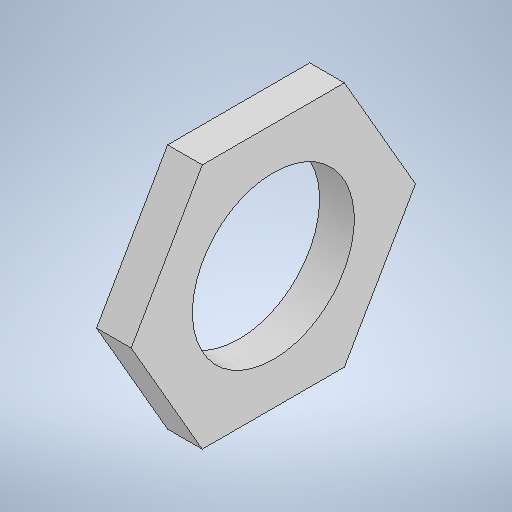
# Autodesk Inventor part: CH-2(Gearbox_Output_Spacer)
Saved by Autodesk Inventor 2025.1 (Build 291241020, 241B)
## iProperties
Created: 2024-10-02
Part Number: CH-2(Gearbox_Output_Spacer)
Material: Generic
Document SubType Name: Modeling
Designer: aidan
Density: 1 g/cm^3
Appearance: Default
Author: aidan
Autodesk Inventor part; units mm, degrees
ref_plane "YZ Plane" through (0, 0, 0) normal (1, 0, 0) x (0, 1, 0)
ref_plane "XZ Plane" through (0, 0, 0) normal (0, 1, 0) x (-1, 0, 0)
ref_plane "XY Plane" through (0, 0, 0) normal (0, 0, 1) x (1, 0, 0)
sketch "Sketch1" plane through (0, 0, 0) normal (1, 0, 0) x (0, 1, 0)
  circle A0 centre (0, 0) radius 7.112
  circle A1 centre (0, 0) radius 12.7
  line L0 (10.8193, 6.6508) -> (10.8193, -6.6508)
  line L1 (-0.3501, 12.6952) -> (11.1694, 6.0444)
  line L2 (-11.1694, 6.0444) -> (0.3501, 12.6952)
  line L3 (-10.8193, -6.6508) -> (-10.8193, 6.6508)
  line L4 (0.3501, -12.6952) -> (-11.1694, -6.0444)
  line L5 (11.1694, -6.0444) -> (-0.3501, -12.6952)
  point P0 (0, -12.4931)
  point P1 (10.8193, -6.2465)
  point P2 (10.8193, 6.2465)
  point P3 (0, 12.4931)
  point P4 (-10.8193, 6.2465)
  point P5 (-10.8193, -6.2465)
  dimension "d0" = 14.224
  dimension "d1" = 25.4
  dimension "d6" = 360
  constraints: 12 end point, 2 centre point, 2 coincident, 2 point on circle, 1 vertical, 19 other
  measures "d0" diameter of A0
  measures "d1" diameter of A1
extrude "Extrusion2" add sketch "Sketch1" along normal blind 3.048 contours L0 L5 L4 L3 L2 L1
body "Solid2"
